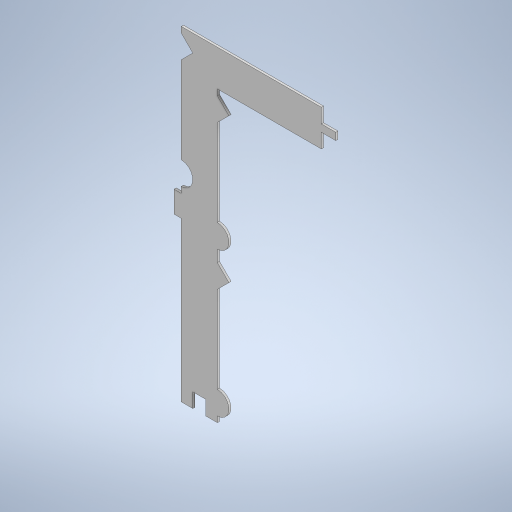
# Autodesk Inventor part: MS_FO_v3
Saved by Autodesk Inventor 2024 (Build 280153000, 153)
## iProperties
Created: 2023-03-29
Part Number: MS_FO_v3
Material: Generic
Document SubType Name: Modeling
Designer: LKLM8608
Density: 1 g/cm^3
Appearance: Default
Author: LKLM8608
Autodesk Inventor part; units mm, degrees
ref_plane "YZ Plane" through (0, 0, 0) normal (1, 0, 0) x (0, 1, 0)
ref_plane "XZ Plane" through (0, 0, 0) normal (0, 1, 0) x (-1, 0, 0)
ref_plane "XY Plane" through (0, 0, 0) normal (0, 0, 1) x (1, 0, 0)
sketch "Sketch1" plane through (0, 0, 0) normal (0, 0, 1) x (1, 0, 0)
  circle A0 centre (-72, 68) radius 8 construction
  line L0 (-72, 76) -> (-64, 68)
  line L1 (-72, 60) -> (-64, 68)
  line L2 (-72, 0) -> (-72, 60)
  line L3 (-72, 76) -> (-72, 80.1)
  line L4 (32, 0) -> (-122.6253, 0) construction
  line L5 (-72, 80.1) -> (0, 80.1)
  line L6 (-72, 0) -> (-72, -8) construction
  arc A1 (-72, -16) -> (-72, 0) centre (-72, -8) ccw
  line L7 (-72, -16) -> (-72, -24.1)
  line L8 (0, 80.1) -> (0, 90.1)
  line L9 (0, 90.1) -> (10, 90.1)
  line L10 (10, 90.1) -> (10, 95.1)
  line L11 (10, 95.1) -> (0, 95.1)
  line L12 (0, 95.1) -> (0, 105.1)
  line L13 (0, 105.1) -> (-97, 105.1)
  line L14 (-72, -120.1) -> (-72, -116.1)
  line L15 (-72, -24.1) -> (-72, -32.1) construction
  arc A2 (-72, -116.1) -> (-72, -100.1) centre (-72, -108.1) ccw
  line L16 (-72, -40.1) -> (-72, -100.1)
  line L17 (-72, -24.1) -> (-64, -32.1)
  line L18 (-64, -32.1) -> (-72, -40.1)
  line L19 (-97, -120.1) -> (-89, -120.1)
  line L20 (-89, -120.1) -> (-89, -110.1)
  line L21 (-89, -110.1) -> (-80, -110.1)
  line L22 (-80, -110.1) -> (-80, -120.1)
  line L23 (-97, -120.1) -> (-89, -120.1)
  line L24 (-80, -120.1) -> (-72, -120.1)
  circle A3 centre (-72, -32.1) radius 8 construction
  line L25 (-64, 68) -> (-64, -32.1) construction
  line L26 (-97, 101.1) -> (-89, 93.1)
  line L27 (-89, 93.1) -> (-97, 85.1)
  arc A4 (-97, 9.1) -> (-97, 25.1) centre (-97, 17.1) ccw
  line L28 (-97, 5) -> (-102, 5)
  line L29 (-102, 5) -> (-102, -10)
  line L30 (-102, -10) -> (-97, -10)
  line L31 (-97, 105.1) -> (-97, 101.1)
  line L32 (-97, 85.1) -> (-97, 25.1)
  line L33 (-97, 9.1) -> (-97, 5)
  line L34 (-97, -10) -> (-97, -120.1)
  circle A5 centre (-97, 93.1) radius 8 construction
  point P0 (0, 0)
  dimension "d5" = 16
  dimension "d132" = 8
  dimension "d162" = 10
  dimension "d163" = 10
  dimension "d164" = 5
  dimension "d165" = 10
  dimension "d166" = 97
  dimension "d168" = 25
  dimension "d171" = 4.1
  dimension "d177" = 8
  dimension "d178" = 10
  dimension "d179" = 9
  dimension "d182" = 76
  dimension "d183" = 72
  dimension "d184" = 80.1
  dimension "d185" = 24.1
  dimension "d186" = 76
  dimension "d187" = 8
  dimension "d188" = 25
  dimension "d189" = 76
  dimension "d190" = 4
  dimension "d191" = 15
  dimension "d192" = 5
  constraints: 70 end point, 23 perpendicular, 9 point on circle, 8 vertical, 6 collinear, 6 equal length, 5 vertical alignment, 4 centre point, 4 horizontal, 3 horizontal alignment, 3 point on line, 2 coincident, 2 equal radius, 1 parallel, 1 tangent, 6 other
  measures "d5" diameter of A0
  measures "d132" distance of L2.start L6.end
  measures "d162" distance of L5.end L8.end
  measures "d163" distance of L8.end L9.end
  measures "d164" distance of L9.end L10.end
  measures "d165" distance of L11.end L12.end
  measures "d166" distance of L12.end L13.end
  measures "d168" distance of L19.start L14.start
  measures "d171" distance of L3.end L0.start
  measures "d177" distance of L19.start L19.end
  measures "d178" distance of L19.end L20.end
  measures "d179" distance of L20.end L21.end
  measures "d182" distance of L6.end A0.centre
  measures "d183" distance between parallel lines of L3 L8
  measures "d184" distance from line of L4.start L5
  measures "d185" distance of L15.end L6.end
  measures "d186" distance of A2.centre L15.end
  measures "d187" distance between parallel lines of L2 L25
  measures "d188" distance between parallel lines of L5 L13
  measures "d189" distance of A4.centre point (-97, 93.1)
  measures "d190" distance of L13.end L26.start
  measures "d191" distance of L28.end L29.end
  measures "d192" distance between parallel lines of L29 L34
extrude "Extrusion10" add sketch "Sketch1" along normal blind 1.5
body "Solid2"
